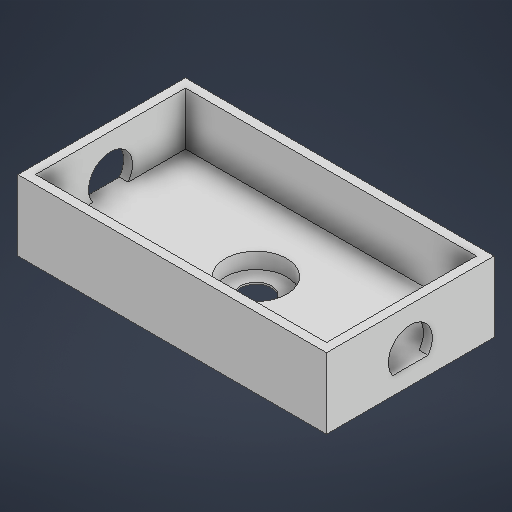
# Autodesk Inventor part: Battery_box
Saved by Autodesk Inventor 2027 (Build 310192060, 192F)
## iProperties
Created: 2026-06-27
Part Number: Battery_box
Material: Ogólny
Document SubType Name: Modeling
Designer: User
Density: 1 g/cm^3
Appearance: Domyślna
Author: User
Autodesk Inventor part; units mm, degrees
ref_plane "YZ Plane" through (0, 0, 0) normal (1, 0, 0) x (0, 1, 0)
ref_plane "XZ Plane" through (0, 0, 0) normal (0, 1, 0) x (-1, 0, 0)
ref_plane "XY Plane" through (0, 0, 0) normal (0, 0, 1) x (1, 0, 0)
sketch "Szkic1" plane through (0, 0, 0) normal (0, 1, 0) x (-1, 0, 0)
  line L0 (-16.5, 8.5) -> (16.5, 8.5)
  line L1 (16.5, 8.5) -> (16.5, -8.5)
  line L2 (16.5, -8.5) -> (-16.5, -8.5)
  line L3 (-16.5, -8.5) -> (-16.5, 8.5)
  line L4 (-16.5, 8.5) -> (16.5, -8.5) construction
  line L5 (16.5, 8.5) -> (-16.5, -8.5) construction
  line L6 (-17.5, 9.5) -> (17.5, 9.5)
  line L7 (17.5, 9.5) -> (17.5, -9.5)
  line L8 (17.5, -9.5) -> (-17.5, -9.5)
  line L9 (-17.5, -9.5) -> (-17.5, 9.5)
  line L10 (-17.5, 9.5) -> (17.5, -9.5) construction
  line L11 (17.5, 9.5) -> (-17.5, -9.5) construction
  circle A0 centre (0, 0) radius 1.75
  circle A1 centre (0, 0) radius 3.5
  dimension "d0" = 33
  dimension "d1" = 17
  dimension "d2" = 35
  dimension "d3" = 19
  dimension "d4" = 3.5
  dimension "d5" = 7
  constraints: 24 end point, 4 midpoint, 4 parallel, 2 centre point, 2 coincident, 2 horizontal, 2 perpendicular
  measures "d0" distance of L1.end L2.end
  measures "d1" distance of L0.end L1.end
  measures "d2" distance of L7.end L8.end
  measures "d3" distance of L6.end L7.end
  measures "d4" diameter of A0
  measures "d5" diameter of A1
extrude "Wyciągnięcie proste1" add sketch "Szkic1" along normal blind 6 contours L6 L7 L8 L9
extrude "Wyciągnięcie proste2" add sketch "Szkic1" against normal blind 2 contours L0 L1 L2 L3 | L6 L7 L8 L9 | A1
extrude "Wyciągnięcie proste3" cut sketch "Szkic1" against normal blind 1.8 contours A1
sketch "Szkic2" plane through (17.5, 6, 9.5) normal (1, 0, 0) x (0, 0, -1)
  line L0 (1, -6) -> (1, 0) projected
  line L1 (18, -6) -> (1, -6) projected
  line L2 (1, -6) -> (18, -6)
  line L3 (9.5, -6) -> (9.5, 0)
  line L4 (0, 0) -> (19, 0) projected
  line L5 (9.5, -6) -> (9.5, -3)
  circle A0 centre (9.5, -4.5) radius 2.5
  point P0 (11.5, -6)
  point P1 (7.5, -6)
  dimension "d14" = 5
  constraints: 6 end point, 3 midpoint, 1 centre point, 1 horizontal
  measures "d14" diameter of A0
extrude "Wyciągnięcie proste4" cut sketch "Szkic2" against normal blind 39.25 contours A0 L3 L1 | L3 A0 L1
